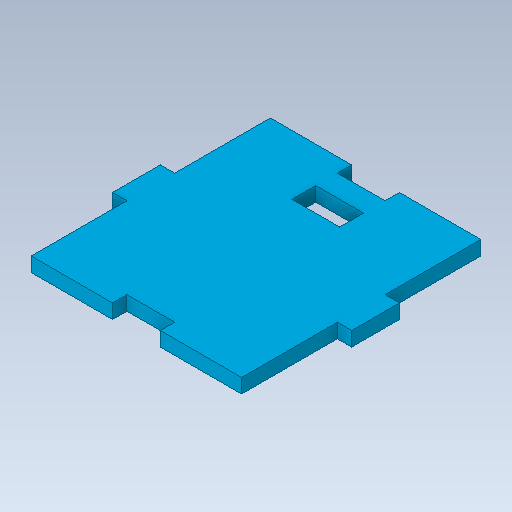
# Autodesk Inventor part: Part9
Saved by Autodesk Inventor 2020 (Build 240168000, 168)
## iProperties
Created: 2020-03-11
Part Number: Part9
Material: Generic
Document SubType Name: Modeling
Designer: tor16003
Density: 1 g/cm^3
Appearance: Sky Blue Medium
Author: tor16003
Autodesk Inventor part; units mm, degrees
ref_plane "YZ Plane" through (0, 0, 0) normal (1, 0, 0) x (0, 1, 0)
ref_plane "XZ Plane" through (0, 0, 0) normal (0, 1, 0) x (-1, 0, 0)
ref_plane "XY Plane" through (0, 0, 0) normal (0, 0, 1) x (1, 0, 0)
sketch "Sketch1" plane through (0, 0, 0) normal (0, 1, 0) x (-1, 0, 0)
  line L0 (44, 0) -> (44, -20)
  line L1 (44, -20) -> (47, -20)
  line L2 (47, -20) -> (47, -30)
  line L3 (47, -30) -> (44, -30)
  line L4 (44, -30) -> (44, -50)
  line L5 (44, -50) -> (27, -50)
  line L6 (27, -50) -> (27, -47)
  line L7 (27, -47) -> (17, -47)
  line L8 (17, -47) -> (17, -50)
  line L9 (17, -50) -> (0, -50)
  line L10 (0, -50) -> (0, -30)
  line L11 (0, -30) -> (-3, -30)
  line L12 (-3, -30) -> (-3, -20)
  line L13 (-3, -20) -> (0, -20)
  line L14 (0, -20) -> (0, 0)
  line L15 (44, 0) -> (27, 0)
  line L16 (27, 0) -> (27, -3)
  line L17 (27, -3) -> (17, -3)
  line L18 (17, -3) -> (17, 0)
  line L19 (17, 0) -> (0, 0)
  line L20 (27, -42.5) -> (17, -42.5)
  line L21 (17, -42.5) -> (17, -37.5)
  line L22 (17, -37.5) -> (27, -37.5)
  line L23 (27, -37.5) -> (27, -42.5)
  point P0 (47, -25)
  point P1 (22, -3)
  point P2 (22, -47)
  point P3 (22, -42.5)
  dimension "d0" = 3
  dimension "d1" = 10
  dimension "d2" = 3
  dimension "d3" = 50
  dimension "d4" = 10
  dimension "d5" = 50
  dimension "d7" = 10
  dimension "d8" = 5
  dimension "d9" = 4.5
  constraints: 48 end point, 16 perpendicular, 7 equal length, 4 horizontal, 4 midpoint, 3 collinear, 3 point on line, 2 coincident, 2 parallel, 1 vertical, 1 vertical alignment
  measures "d0" distance of L7.end L8.end
  measures "d1" distance of L1.end L2.end
  measures "d2" distance of L0.end L1.end
  measures "d3" distance between parallel lines of L12 L2
  measures "d4" distance of L6.end L7.end
  measures "d5" distance between parallel lines of L19 L9
  measures "d7" distance of L21.end L22.end
  measures "d8" distance of L20.end L21.end
  measures "d9" distance between parallel lines of L7 L20
extrude "Extrusion1" add sketch "Sketch1" along normal blind 3
body "Solid1"
